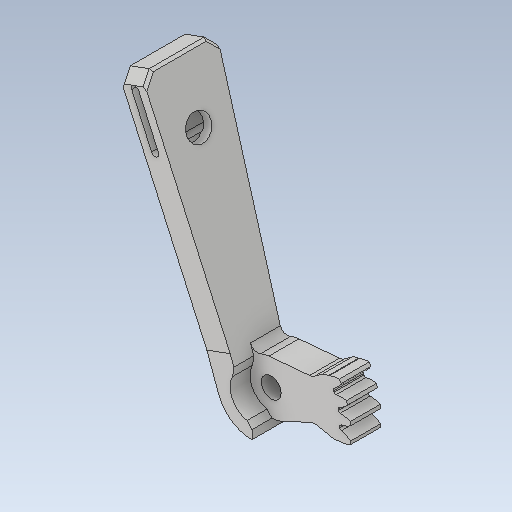
# Autodesk Inventor part: Gimbal_Hebel_links
Saved by Autodesk Inventor 2021 (Build 250183000, 183)
## iProperties
Created: 2020-05-23
Part Number: Gimbal_Hebel_links
Material: Polylactid (PLA)
Document SubType Name: Modeling
Designer: Alex
Density: 1.3 g/cm^3
Appearance: Generisch
Mass: 5.10712 g
Surface Area: 29.6415 cm^2
Volume: 3.92856 cm^3
Author: Alex
Autodesk Inventor part; units mm, degrees
ref_plane "Skizzenebene Hebel_links" through (-3.7986, -3.748, 5) normal (0, 0, 1) x (1, 0, 0)
ref_plane "Erhebung Hilfsebene" through (-24.5556, 61.4336, 7.3001) normal (-0.3420201, 0.9396926, 0) x (-0.9396926, -0.3420201, 0)
ref_plane "Skizzenebene_Hebelarm" through (-3.2669, 0, 5) normal (0, 0, 1) x (1, 0, 0)
sketch "Skizze1" plane through (0, 0, 0) normal (0, 0, 1) x (1, 0, 0)
  circle A0 centre (-3.9903, 14) radius 4 construction
  circle A1 centre (-3.9903, 14) radius 5.25 construction
  line L0 (-1.7715, 9.2419) -> (4.5427, 12.1863)
  line L1 (-1.8481, 4) -> (24.1519, 4) construction
  line L2 (-4.4485, 19.23) -> (4.258, 19.9927)
  arc A2 (-4.4485, 19.23) -> (-1.7715, 9.2419) centre (-3.9903, 14) ccw
  line L3 (-0.7542, 16.3511) -> (7.1337, 22.082)
  arc A3 (7.2017, 21.9877) -> (7.1337, 22.082) centre (-3.9903, 14) ccw
  arc A4 (7.2017, 21.9877) -> (7.665, 21.861) centre (7.511, 22.2084) ccw
  arc A5 (9.6881, 22.3008) -> (7.665, 21.861) centre (9.7439, 17.1708) ccw
  arc A6 (10.0376, 21.6954) -> (9.6881, 22.3008) centre (-3.9903, 14) ccw
  arc A7 (8.6452, 20.1632) -> (10.0376, 21.6954) centre (5.6228, 24.3087) ccw
  arc A8 (8.6452, 20.1632) -> (8.5232, 19.6987) centre (8.869, 19.8562) ccw
  arc A9 (8.6178, 19.4862) -> (8.5232, 19.6987) centre (-3.9903, 14) ccw
  arc A10 (8.6178, 19.4862) -> (9.0447, 19.266) centre (8.9663, 19.6378) ccw
  arc A11 (11.115, 19.2755) -> (9.0447, 19.266) centre (10.103, 14.246) ccw
  arc A12 (11.331, 18.6107) -> (11.115, 19.2755) centre (-3.9903, 14) ccw
  arc A13 (9.6505, 17.4015) -> (11.331, 18.6107) centre (7.556, 22.0848) ccw
  arc A14 (9.6505, 17.4015) -> (9.4346, 16.9725) centre (9.8056, 17.0546) ccw
  arc A15 (9.483, 16.7449) -> (9.4346, 16.9725) centre (-3.9903, 14) ccw
  arc A16 (9.483, 16.7449) -> (9.8547, 16.4408) centre (9.8553, 16.8208) ccw
  arc A17 (11.8817, 16.0196) -> (9.8547, 16.4408) centre (9.8461, 11.3105) ccw
  arc A18 (11.9548, 15.3245) -> (11.8817, 16.0196) centre (-3.9903, 14) ccw
  arc A19 (10.0596, 14.4911) -> (11.9548, 15.3245) centre (8.9846, 19.5075) ccw
  arc A20 (10.0596, 14.4911) -> (9.7592, 14.1163) centre (10.1392, 14.1195) ccw
  arc A21 (9.7592, 13.8837) -> (9.7592, 14.1163) centre (-3.9903, 14) ccw
  arc A22 (9.7592, 13.8837) -> (10.0596, 13.5089) centre (10.1392, 13.8805) ccw
  arc A23 (11.9548, 12.6755) -> (10.0596, 13.5089) centre (8.9846, 8.4925) ccw
  arc A24 (11.8817, 11.9804) -> (11.9548, 12.6755) centre (-3.9903, 14) ccw
  arc A25 (9.8547, 11.5592) -> (11.8817, 11.9804) centre (9.8461, 16.6895) ccw
  arc A26 (9.8547, 11.5592) -> (9.483, 11.2551) centre (9.8553, 11.1792) ccw
  arc A27 (9.4593, 11.1412) -> (9.483, 11.2551) centre (-3.9903, 14) ccw
  line L4 (9.4593, 11.1412) -> (-0.0777, 13.1684)
  arc A28 (-0.0777, 13.1684) -> (-0.7542, 16.3511) centre (-3.9903, 14) ccw
  spline S0 degree 3 poles (-0.8481, 20.5) (-0.8481, 20.4398) (-0.8631, 20.3692) (-0.912, 20.2565) (-0.9555, 20.1951) (-1.0485, 20.1065) (-1.1152, 20.0644) (-1.2397, 20.0151) (-1.32, 20) (-1.3881, 20) knots 0 0 0 0 0.234395 0.234395 0.478664 0.478664 0.734739 0.734739 1 1 1 1
  circle A29 centre (-3.9903, 14) radius 2
  dimension "d0" = 10.5
  dimension "d1" = 8
  dimension "d2" = 25
  dimension "d46" = 0.5
  constraints: 4 end point, 4 point on circle, 4 tangent, 3 centre point, 2 point on line, 1 coincident, 1 concentric
  measures "d0" diameter of A1
  measures "d1" diameter of A0
  measures "d2" angle of L1 L0
  measures "d46" distance from line of L2 point (-1.388, 20)
extrude "Stirnverzahnung" add sketch "Skizze1" along normal blind 6 contours A2 L2 L3 A28 L4 L0 | L4 A28 L3 A3 A4 A5 A6 A7 A8 A9 A10 A11 A12 A13 A14 A15 A16 A17 A18 A19 A20 A21 A22 A23 A24 A25 A26 A27 | A29
sketch "Skizze2" plane through (-3.7986, -3.748, 5) normal (0, 0, 1) x (1, 0, 0)
  arc A0 (-6.7695, 15.3539) -> (-0.0495, 10.7495) centre (-0.1916, 17.748) ccw
  line L0 (-6.7695, 15.3539) -> (-9.1137, 21.7946)
  line L1 (-9.1137, 21.7946) -> (-4.4153, 23.5047)
  line L2 (-4.4153, 23.5047) -> (-3.7312, 21.6254)
  arc A1 (-3.7312, 21.6254) -> (-0.0495, 12.4999) centre (-0.1916, 17.748) ccw
  line L3 (-0.0495, 12.4999) -> (-0.0495, 10.7495)
  arc A2 (-0.6498, 22.978) -> (2.0271, 12.9899) centre (-0.1916, 17.748) ccw construction
  line L4 (14.9505, 0.0367) -> (14.9505, 27.4161) construction
  line L5 (-0.0495, 3.948) -> (-0.0495, 11.248) construction
  dimension "d26" = 5
  dimension "d27" = 10.5
  dimension "d28" = 14
  dimension "d29" = 2
  dimension "d39" = 20
  constraints: 8 end point, 4 point on circle, 2 centre point, 2 tangent, 1 collinear, 1 concentric, 1 perpendicular
  measures "d26" distance between parallel lines of L2 L0
  measures "d27" diameter of A1
  measures "d28" diameter of A0
  measures "d29" distance of L1.end L2.end
  measures "d39" angle of L4 L2
extrude "Hebelarm_basis" add sketch "Skizze2" along normal mid plane 10
fillet "Konturverrundung:1" radius 2 4 edges at (4.5427, 12.1863, 3) (9.4593, 11.1412, 3) (4.258, 19.9927, 3) (7.1337, 22.082, 3)
sketch "Skizze3" plane through (-12.9124, 18.0466, 10) normal (-0.3420201, 0.9396926, 0) x (0.9396926, 0.3420201, 0)
  line L0 (0, 10) -> (0, 0) projected
  line L1 (5, 0) -> (0, 0) projected
  line L2 (5, 10) -> (5, 0) projected
  line L3 (0, 10) -> (5, 10) projected
  point P0 (5.9613, 10)
sketch "Skizze4" plane through (-24.5556, 61.4336, 7.3001) normal (-0.3420201, 0.9396926, 0) x (-0.9396926, -0.3420201, 0)
  line L0 (-4.46, -7.3001) -> (-4.46, -7.3001) construction
  line L1 (3.8982, -7.3001) -> (3.8982, 2.6999) construction
  line L2 (3.8982, -7.3001) -> (-1.1018, 2.6999) construction
  line L3 (-1.1018, -7.3001) -> (-1.1018, -7.3001) construction
  line L4 (-1.1018, -7.3001) -> (3.8982, 2.6999) construction
  line L5 (3.8982, -9.8001) -> (-1.1018, -9.8001)
  line L6 (-1.1018, -9.8001) -> (-1.1018, 5.1999)
  line L7 (-1.1018, 5.1999) -> (3.8982, 5.1999)
  line L8 (3.8982, 5.1999) -> (3.8982, -9.8001)
  line L9 (3.8982, -9.8001) -> (-1.1018, 5.1999) construction
  line L10 (-1.1018, -9.8001) -> (3.8982, 5.1999) construction
  point P0 (1.3982, -2.3001)
  dimension "d30" = 15
  constraints: 16 end point, 3 midpoint, 2 parallel, 1 collinear, 1 horizontal, 1 horizontal alignment, 1 perpendicular
  measures "d30" distance of L7.end L5.start
loft "Hebelarm" add profiles "Skizze3", "Skizze4"
fillet "Konturverrundung:2" radius 1.5 1 edges at (-7.5299, 17.8773, 3)
chamfer "Konturfase:1" distance 2 angle 45 2 edges at (-25.8694, 60.9554, 12.5) (-25.8694, 60.9554, -2.5)
chamfer "Konturfase:2" distance 0.5 angle 45 6 edges at (-27.8772, 59.1621, 11.4442) (-23.1787, 60.8722, 11.4442) (-23.5202, 61.8104, 5) (-28.2187, 60.1003, 5) (-27.8772, 59.1621, -1.4442) (-23.1787, 60.8722, -1.4442)
sketch "Skizze5" plane through (-3.2669, 0, 6) normal (0, 0, 1) x (1, 0, 0)
  line L0 (-22.6025, 60.9554) -> (-17.9863, 48.2724) construction
  line L1 (-21.663, 58.3741) -> (-18.2428, 48.9772) construction
  line L2 (-20.9583, 58.6306) -> (-17.5381, 49.2337)
  line L3 (-18.9476, 48.7207) -> (-22.3678, 58.1176)
  arc A0 (-20.9583, 58.6306) -> (-22.3678, 58.1176) centre (-21.663, 58.3741) ccw
  arc A1 (-18.9476, 48.7207) -> (-17.5381, 49.2337) centre (-18.2428, 48.9772) ccw
  line L4 (-20.0402, 59.7629) -> (-23.7989, 58.3949) construction
  line L5 (-24.4819, 60.2713) -> (-20.7231, 61.6394) construction
  point P0 (3.2669, 0)
  point P1 (-19.9529, 53.6757)
  dimension "d22" = 1.5
  dimension "d23" = 10
  constraints: 10 end point, 5 point on circle, 5 tangent, 2 centre point, 2 midpoint, 2 point on line, 1 parallel, 1 perpendicular
  measures "d22" distance between parallel lines of L3 L2
  measures "d23" distance of L1.end L1.start
extrude "Klettverschlussaufnahme" cut sketch "Skizze5" along normal through all both and the other way through all
sketch "Skizze6" plane through (0, 0, 6) normal (0, 0, 1) x (1, 0, 0)
  circle A0 centre (-3.9903, 14) radius 1.7 projected
  point P0 (0, 0)
  point P1 (-3.9903, 14)
  constraints: 1 coincident
hole "Einfach_Keine_4 mm" at (-3.9903, 14, 6) direction (0, 0, -1) diameter 4 end through all
sketch "Skizze7" plane through (-3.7986, -3.748, 10) normal (0, 0, 1) x (1, 0, 0)
  circle A0 centre (-0.1916, 17.748) radius 4.2505 construction
  arc A1 (-0.6498, 22.978) -> (-2.3477, 22.5348) centre (-0.1916, 17.748) ccw construction
  line L0 (-0.0495, 12.4999) -> (-0.0495, 13.4999)
  line L1 (-3.7312, 21.6254) -> (-4.4153, 23.5047) construction
  line L2 (-3.7312, 21.6254) -> (-3.3538, 20.5883)
  arc A2 (-3.3538, 20.5883) -> (-0.0495, 13.4999) centre (-0.1916, 17.748) ccw
  arc A3 (-3.7312, 21.6254) -> (-0.0495, 12.4999) centre (-0.1916, 17.748) ccw
  circle A4 centre (-0.1916, 17.748) radius 2 projected
  point P0 (3.7986, 3.748)
  point P1 (2.0271, 12.9899)
  dimension "d40" = 1
  constraints: 6 point on circle, 4 end point, 3 centre point, 2 concentric, 1 coincident, 1 collinear, 1 vertical
  measures "d40" distance of L0.start L0.end
extrude "Nachbearbeitung: Auflagefläche" add sketch "Skizze7" against normal up to surface (4 mm away) contours A3 L2 A2 L0
chamfer "Fase3" distance 1 angle 45 2 edges at (-3.8481, 9.7519, 8) (-7.1524, 16.8403, 8)
sketch "Skizze8" plane through (-8.172, 19.6415, 6) normal (0.9396926, 0.3420201, 0) x (0, 0, -1)
  line L0 (8.7, -8.7315) -> (8.7, -4.7315) construction
  line L1 (-6.7, -4.7315) -> (-6.7, -8.7315) construction
  line L2 (8.7, -6.7315) -> (-6.7, -6.7315) construction
  circle A0 centre (1, 33.2685) radius 2.5
  line L3 (1, -40.0322) -> (1, 60.6456) projected
  point P0 (6, -21.2519)
  dimension "d47" = 40
  dimension "d48" = 5
  constraints: 2 end point, 2 midpoint, 1 centre point, 1 point on line
  measures "d47" distance from line of L2 A0.centre
  measures "d48" diameter of A0
extrude "Extrusion5" cut sketch "Skizze8" against normal blind 2
